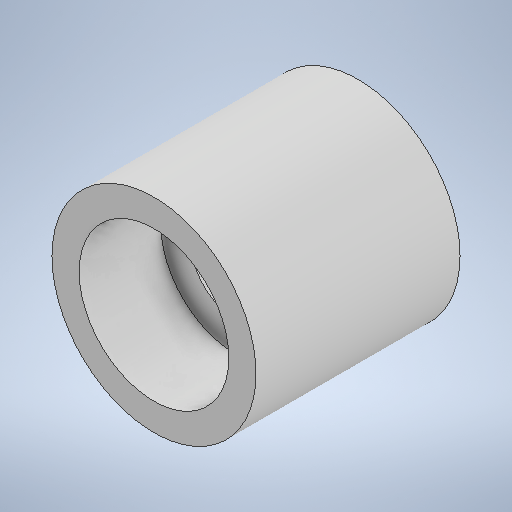
# Autodesk Inventor part: sroub_dira
Saved by Autodesk Inventor 2025 (Build 290162000, 162)
## iProperties
Created: 2024-12-13
Part Number: sroub_dira
Material: Všeobecné
Document SubType Name: Modeling
Designer: lukas
Density: 1 g/cm^3
Appearance: Výchozí
Author: lukas
## iProperties of the stored document sroub_dira_3D tisk.ipt
Created: 2024-12-13
Part Number: sroub_dira_3D tisk
Material: Všeobecné
Document SubType Name: Modeling
Designer: lukas
Density: 1 g/cm^3
Appearance: Výchozí
Author: lukas
Autodesk Inventor part; units mm, degrees
ref_plane "YZ Plane" through (0, 0, 0) normal (1, 0, 0) x (0, 1, 0)
ref_plane "XZ Plane" through (0, 0, 0) normal (0, 1, 0) x (-1, 0, 0)
ref_plane "XY Plane" through (0, 0, 0) normal (0, 0, 1) x (1, 0, 0)
sketch "Náčrt1" plane through (0, 0, 0) normal (0, 0, 1) x (1, 0, 0)
  line L0 (-10.5, 0) -> (10.5, 0) projected
  line L1 (0, -10.5) -> (0, 10.5) projected
  circle A0 centre (0, 0) radius 7.5
  dimension "d9" = 15
  constraints: 1 centre point, 1 coincident
  measures "d9" diameter of A0
extrude "Vysunutí1" add sketch "Náčrt1" along normal blind 15
sketch "Náčrt2" plane through (0, 0, 15) normal (0, 0, 1) x (1, 0, 0)
  circle A0 centre (0, 0) radius 7.5 projected
  constraints: 1 coincident
hole "Díra1" at (0, 0, 15) direction (0, 0, -1) diameter 6.6 end through all counterbore diameter 11 counterbore depth 6 clearance for "Strojní šroub se zápustnou hlavou" size "M6" standard "Ansi M metrický profil"
